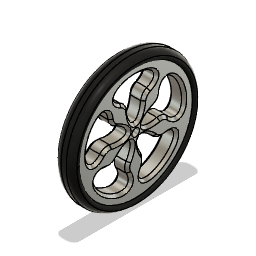
SternradGenerativeDesign (Autodesk Fusion 360 archive; units mm, degrees)
design "Rad"
Autodesk Fusion 360 part; units mm, degrees
cylinder "Grundkörper Zylinder1" add diameter 250 height 40 placed x (0, 0, -1) y (0, 1, 0) z (1, 0, 0) at (0, 25, 0) makes body 1
move_body "Verschieben1" bodies 1 to x (1, 0, 0) y (0, 1, 0) z (0, 0, 1) at (0, 100, 0)
copy_body "Körper kopieren/einfügen1" bodies 1 makes body 2
move_body "Verschieben2" bodies 2 to x (1, 0, 0) y (0, 1, 0) z (0, 0, 1) at (0, 0, -280)
copy_body "Körper kopieren/einfügen2" bodies 1 makes body 3
move_body "Verschieben3" bodies 3 to x (1, 0, 0) y (0, 0.866025, -0.5) z (0, 0.5, 0.866025) at (0, 259.2339, -77.5)
delete_body "Körper entfernen1" bodies 2
delete_body "Körper entfernen2" bodies 3
fillet "Abrundung1" radius 15 2 edges at (40, 79.7981, 116.5409) (0, 170.2019, 116.5409) on bodies 1
extrude "Extrusion1" cut 1 faces at (40, 142.8595, -12.1764) along direction (-1, 0, 0) blind 5 on bodies 1 bodies 1
extrude "Extrusion2" cut 1 faces at (0, 142.8595, -12.1764) along direction (1, 0, 0) blind 5 on bodies 1 bodies 1
fillet "Abrundung2" radius 5 2 edges at (0, 164.7777, -102.556) (40, 85.2223, -102.556) on bodies 1
sketch "Skizze2" plane through (5, 0, 0) normal (-1, 0, 0) x (0, 0, 1)
  circle A0 centre (0, 125) radius 110
  line L0 (0, 125) -> (0, 235)
  line L1 (0, 180) -> (0, 220)
  ellipse E0 centre (0, 180) end of major axis (0, 220) minor radius 15 (-14.3969, 168.7714) -> (14.3969, 168.7714) ccw
  ellipse E1 centre (0, 200) end of major axis (-40, 200) minor radius 20 (26.2858, 184.9247) -> (-26.2858, 184.9247) ccw
  arc A1 (-14.3969, 168.7714) -> (-26.2858, 184.9247) centre (-34.2776, 166.5909) ccw
  arc A2 (26.2858, 184.9247) -> (14.3969, 168.7714) centre (34.2776, 166.5909) ccw
  arc A3 (-46.0779, 124.8339) -> (-65.1145, 118.5185) centre (-50.1476, 105.2523) ccw
  ellipse E2 centre (-71.3292, 148.1763) end of major axis (-83.6899, 110.134) minor radius 20 (-48.869, 168.517) -> (-65.1145, 118.5185) ccw
  arc A4 (-48.869, 168.517) -> (-37.1802, 152.2183) centre (-28.9629, 170.4523) ccw
  ellipse E3 centre (-52.3081, 141.9959) end of major axis (-90.3504, 154.3566) minor radius 15 (-46.0779, 124.8339) -> (-37.1802, 152.2183) ccw
  arc A5 (-14.0808, 81.126) -> (-13.9572, 61.0695) centre (3.2847, 71.2044) ccw
  ellipse E4 centre (-44.0839, 64.3237) end of major axis (-11.7232, 40.8123) minor radius 20 (-56.4885, 91.9703) -> (-13.9572, 61.0695) ccw
  arc A6 (-56.4885, 91.9703) -> (-37.3755, 98.0505) centre (-52.1777, 111.5002) ccw
  ellipse E5 centre (-32.3282, 80.5041) end of major axis (-55.8396, 48.1434) minor radius 15 (-14.0808, 81.126) -> (-37.3755, 98.0505) ccw
  arc A7 (37.3755, 98.0505) -> (56.4885, 91.9703) centre (52.1777, 111.5002) ccw
  ellipse E6 centre (44.0839, 64.3237) end of major axis (76.4446, 87.8351) minor radius 20 (13.9572, 61.0695) -> (56.4885, 91.9703) ccw
  arc A8 (13.9572, 61.0695) -> (14.0808, 81.126) centre (-3.2847, 71.2044) ccw
  ellipse E7 centre (32.3282, 80.5041) end of major axis (55.8396, 48.1434) minor radius 15 (37.3755, 98.0505) -> (14.0808, 81.126) ccw
  arc A9 (37.1802, 152.2183) -> (48.869, 168.517) centre (28.9629, 170.4523) ccw
  ellipse E8 centre (71.3292, 148.1763) end of major axis (58.9686, 186.2185) minor radius 20 (65.1145, 118.5185) -> (48.869, 168.517) ccw
  arc A10 (65.1145, 118.5185) -> (46.0779, 124.8339) centre (50.1476, 105.2523) ccw
  ellipse E9 centre (52.3081, 141.9959) end of major axis (90.3504, 154.3566) minor radius 15 (37.1802, 152.2183) -> (46.0779, 124.8339) ccw
  dimension "d13" = 40
  dimension "d15" = 360
  constraint coincident A0.centre L0.start
  constraint coincident A0 L0.end
  constraint vertical L0
  constraint midpoint L0 L1.start
  constraint coincident L1.start E0.centre
  constraint midpoint L1 E1.centre
  constraint coincident L1.end E1
  constraint tangent E1 A1
  constraint tangent E0 A1
  constraint symmetric L0 A1.end A2.start
  constraint symmetric L0 A1 A2
  constraint symmetric L0 A1.start A2.end
  measures "d13" diameter of A1
extrude "Extrusion3" cut sketch "Skizze2" against normal blind 60 contours L0 L1 E0 E1 A1 | L0 L1 E0 E1 A2 | A3 E2 A4 E3 | A5 E4 A6 E5 | A7 E6 A8 E7 | A9 E8 A10 E9 bodies 1
chamfer "Fase1" distance 5 angle 45 40 edges at (5, 129.6353, -14.2658) (5, 124.235, -56.4451) (5, 154.3566, -90.3504) (5, 158.7965, -45.2154) (5, 140, 0) (5, 178.4461, -18.1701) (5, 220, 0) (5, 178.4461, 18.1701) (5, 129.6353, 14.2658) (5, 158.7965, 45.2154) (5, 154.3566, 90.3504) (5, 124.235, 56.4451) (5, 112.8647, 8.8168) (5, 92.4413, 46.1147) (5, 48.1434, 55.8396) (5, 71.0811, 16.7149) (5, 112.8647, -8.8168) (5, 71.0811, -16.7149) (5, 48.1434, -55.8396) (5, 92.4413, -46.1147) (35, 112.8647, -8.8168) (35, 92.4413, -46.1147) (35, 48.1434, -55.8396) (35, 71.0811, -16.7149) (35, 71.0811, 16.7149) (35, 48.1434, 55.8396) (35, 92.4413, 46.1147) (35, 112.8647, 8.8168) (35, 124.235, 56.4451) (35, 154.3566, 90.3504) (35, 158.7965, 45.2154) (35, 129.6353, 14.2658) (35, 140, 0) (35, 178.4461, 18.1701) (35, 220, 0) (35, 178.4461, -18.1701) (35, 129.6353, -14.2658) (35, 158.7965, -45.2154) (35, 154.3566, -90.3504) (35, 124.235, -56.4451) on bodies 1
cylinder "Grundkörper Zylinder2" cut diameter 15 height -40 placed x (0, 0, 1) y (0, 1, 0) z (-1, 0, 0) at (5, 125, 0) bodies 1
